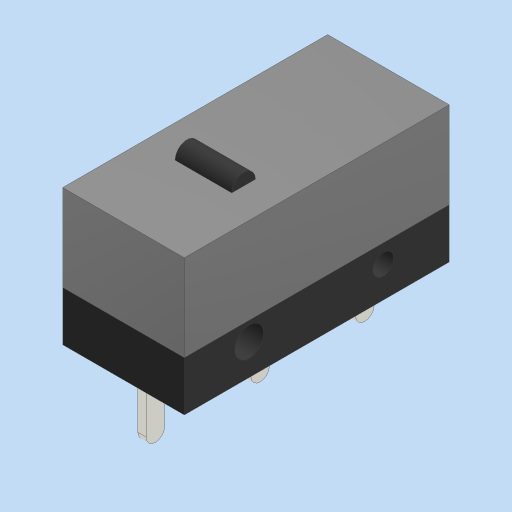
# Autodesk Inventor part: Kailh_GM_8.0_switch
Saved by Autodesk Inventor 2024 (Build 280153000, 153)
## iProperties
Created: 2025-05-06
Part Number: Kailh_GM_8.0_switch
Material: Generic
Document SubType Name: Modeling
Designer: XxPan
Mass: 0.491443 g
Surface Area: 4.65784 cm^2
Volume: 0.491443 cm^3
Density: 1 g/cm^3
Appearance: Default
Author: XxPan
Autodesk Inventor part; units mm, degrees
ref_plane "YZ Plane" through (0, 0, 0) normal (1, 0, 0) x (0, 1, 0)
ref_plane "XZ Plane" through (0, 0, 0) normal (0, 1, 0) x (-1, 0, 0)
sketch "Sketch1" plane through (0, 0, 0) normal (0, 1, 0) x (-1, 0, 0)
  line L0 (2.95, 6.425) -> (-2.95, 6.425)
  line L1 (-2.95, 6.425) -> (-2.95, -6.425)
  line L2 (-2.95, -6.425) -> (2.95, -6.425)
  line L3 (2.95, -6.425) -> (2.95, 6.425)
  line L4 (4.13, 0) -> (-4.13, 0) construction
  line L5 (0, -8.995) -> (0, 8.995) construction
  point P0 (0, 0)
  dimension "d0" = 5.9
  dimension "d1" = 12.85
  constraints: 8 end point, 2 parallel, 1 horizontal, 1 perpendicular, 2 other
  measures "d0" distance of L2.end L1.end
  measures "d1" distance of L1.end L0.end
extrude "Extrusion1" add sketch "Sketch1" along normal blind 6.6
sketch "Sketch2" plane through (2.95, 0, 6.425) normal (1, 0, 0) x (0, 0, -1)
  circle A0 centre (3.15, 1.5) radius 0.7
  circle A1 centre (9.65, 1.5) radius 0.5
  line L0 (0, 0) -> (0, 6.6) projected
  line L1 (0, 0) -> (12.85, 0) projected
  point P0 (6.425, 0)
  dimension "d4" = 1.4
  dimension "d5" = 1
  dimension "d6" = 3.15
  dimension "d7" = 6.5
  dimension "d8" = 1.5
  constraints: 2 centre point, 1 horizontal alignment
  measures "d4" diameter of A0
  measures "d5" diameter of A1
  measures "d6" distance from line of L0 A0.centre
  measures "d7" distance of A1.centre A0.centre
  measures "d8" distance from line of L1 A0.centre
extrude "Extrusion2" cut sketch "Sketch2" against normal through all
sketch "Sketch3" plane through (0, 0, 0) normal (1, 0, 0) x (0, 1, 0)
  line L0 (6.6, -6.425) -> (6.6, 6.425) projected
  circle A0 centre (6.6, 1.975) radius 0.575
  circle A1 centre (1.5, -3.225) radius 0.5 projected
  point P0 (0, 0)
  point P1 (6.6, 2.55)
  point P2 (6.6, 1.4)
  dimension "d11" = 1.15
  dimension "d12" = 5.2
  constraints: 1 centre point, 1 point on line
  measures "d11" diameter of A0
  measures "d12" vertical distance of A1.centre A0.centre
extrude "Extrusion3" add sketch "Sketch3" along normal mid plane 2.75 contours L0 A0 picked at (6.6832, 2.1477)
sketch "Sketch4" plane through (0, 0, 0) normal (1, 0, 0) x (0, 1, 0)
  line L0 (0, 6.425) -> (0, -6.425) projected
  line L1 (0, 0.45) -> (-2.75, 0.45)
  line L2 (0, -0.45) -> (-2.75, -0.45)
  arc A0 (-2.75, 0.45) -> (-2.75, -0.45) centre (-2.75, 0) ccw
  line L3 (-5.275, 0) -> (9.25, 0) construction
  point P0 (0, 0)
  point P1 (-3.2, 0)
  dimension "d15" = 3.2
  dimension "d16" = 0.9
  constraints: 4 end point, 3 point on circle, 2 horizontal, 2 point on line, 2 tangent, 1 centre point, 1 other
  measures "d15" distance from line of point (-3.2, 0) L0
  measures "d16" distance between parallel lines of L2 L1
extrude "Extrusion4" add sketch "Sketch4" along normal mid plane 0.4
pattern_linear "Rectangular Pattern1" count 2 spacing 5.08 along (0, 0, -1) count 2 spacing 5.08 along (0, 0, 1) of "Extrusion4"
ref_plane "Work Plane1" through (0, 2.4, 0) normal (0, 1, 0) x (1, 0, 0)
split_face "Split1"
body "Solid1"
